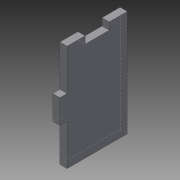
# Autodesk Inventor part: battery holder ends
Saved by Autodesk Inventor 2015 (Build 190159000, 159)
## iProperties
Created: 2014-08-15
Part Number: battery holder ends
Material: Generic
Document SubType Name: Modeling
Designer: karl
Density: 1 g/cm^3
Appearance: Default
Author: karl
Autodesk Inventor part; units mm, degrees
ref_plane "YZ Plane" through (0, 0, 0) normal (1, 0, 0) x (0, 1, 0)
ref_plane "XZ Plane" through (0, 0, 0) normal (0, 1, 0) x (-1, 0, 0)
ref_plane "XY Plane" through (0, 0, 0) normal (0, 0, 1) x (1, 0, 0)
sketch "Sketch1" plane through (0, 0, 0) normal (1, 0, 0) x (0, 1, 0)
  line L0 (-12.5, -22) -> (12.5, -22)
  line L1 (12.5, -22) -> (12.5, 22)
  line L2 (12.5, 22) -> (-12.5, 22)
  line L3 (-12.5, 22) -> (-12.5, -22)
  line L4 (-12.5, -22) -> (12.5, 22) construction
  line L5 (12.5, -22) -> (-12.5, 22) construction
  point P0 (0, 0)
  dimension "d0" = 25
  dimension "d1" = 44
  constraints: 12 end point, 2 midpoint, 2 parallel, 1 horizontal, 1 perpendicular
  measures "d0" distance of L2.end L1.end
  measures "d1" distance of L1.end L0.end
extrude "Extrusion1" add sketch "Sketch1" along normal blind 3
sketch "Sketch2" plane through (0, 0, 0) normal (-1, 0, 0) x (0, 0, 1)
  line L0 (-5, -12.5) -> (5, -12.5)
  line L1 (5, -12.5) -> (5, -15.5)
  line L2 (5, -15.5) -> (-5, -15.5)
  line L3 (-5, -15.5) -> (-5, -12.5)
  line L4 (22, -12.5) -> (-22, -12.5) projected
  point P0 (0, 0)
  point P1 (0, -15.5)
  dimension "d4" = 10
  dimension "d5" = 3
  constraints: 8 end point, 2 parallel, 1 collinear, 1 horizontal, 1 midpoint, 1 perpendicular, 1 vertical alignment
  measures "d4" distance of L1.end L2.end
  measures "d5" distance of L0.end L1.end
extrude "Extrusion2" add sketch "Sketch2" against normal blind 3
sketch "Sketch3" plane through (0, 0, 0) normal (-1, 0, 0) x (0, 0, 1)
  line L0 (22, 12.5) -> (22, -12.5) projected
  line L1 (22, 5) -> (19, 5)
  line L2 (19, 5) -> (19, -5)
  line L3 (19, -5) -> (22, -5)
  line L4 (22, -5) -> (22, 5)
  point P0 (0, 0)
  point P1 (19, 0)
  dimension "d8" = 3
  dimension "d9" = 10
  constraints: 8 end point, 2 parallel, 1 horizontal, 1 horizontal alignment, 1 midpoint, 1 perpendicular, 1 point on line
  measures "d8" distance of L3.end L2.end
  measures "d9" distance of L2.end L1.end
extrude "Extrusion3" cut sketch "Sketch3" against normal blind 3
mirror "Mirror1" about plane through (0, 0, 0) normal (0, 0, 1) of "Extrusion3"
body "Solid1"
